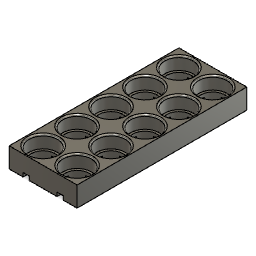
Battery-holder-103.6v-18650 (Autodesk Fusion 360 design; units mm, degrees)
Autodesk Fusion 360 part; units mm, degrees
note: some values were not read from the file. Set by a fixed rule: which sketch regions a step uses.
sketch "Sketch1" plane through (0, 0, 0) normal (0, 1, 0) x (1, 0, 0)
  line L0 (0, 0) -> (-55, 0)
  line L1 (-55, 0) -> (-55, -100.2)
  line L2 (-55, -100.2) -> (0, -100.2)
  line L3 (0, -100.2) -> (0, 0)
  dimension "d1" = 55
  dimension "d2" = 100.2
  constraint horizontal L0
  constraint vertical L1
  constraint horizontal L2
  constraint vertical L3
  constraint coincident L0.start L3.end
  measures "d1" distance of L0.start L0.end
  measures "d2" distance of L0.start L2.end
extrude "Extrude1" add sketch "Sketch1" along normal blind 6
sketch "Sketch2" plane through (0, 6, 0) normal (0, 1, 0) x (-1, 0, 0)
  line L0 (0, 100.2) -> (0, 0)
  line L1 (0, 0) -> (55, 0)
  line L2 (55, 0) -> (55, 100.2)
  line L3 (55, 100.2) -> (0, 100.2)
  circle A0 centre (4, 5) radius 1.5
  circle A1 centre (4, 95.2) radius 1.5
  circle A2 centre (51, 95.2) radius 1.5
  circle A3 centre (51, 5) radius 1.5
  dimension "d13" = 3
  dimension "d14" = 3
  dimension "d15" = 3
  dimension "d16" = 3
  measures "d13" diameter of A0
  measures "d14" diameter of A1
  measures "d15" diameter of A2
  measures "d16" diameter of A3
extrude "Extrude2" cut sketch "Sketch2" against normal blind 6 contours A0 | A1 | A2 | A3
sketch "Sketch3" plane through (0, 6, 0) normal (0, 1, 0) x (-1, 0, 0)
  circle A0 centre (4, 95.2) radius 1.5
  circle A1 centre (51, 5) radius 1.5
  circle A2 centre (51, 95.2) radius 1.5
  circle A3 centre (4, 5) radius 1.5
  line L0 (0, 100.2) -> (0, 0)
  line L1 (0, 0) -> (55, 0)
  line L2 (55, 0) -> (55, 100.2)
  line L3 (55, 100.2) -> (0, 100.2)
  circle A4 centre (4, 95.2) radius 3
  circle A5 centre (51, 95.2) radius 3
  circle A6 centre (4, 5) radius 3
  circle A7 centre (51, 5) radius 3
  dimension "d19" = 1.5
  dimension "d20" = 1.5
  dimension "d21" = 1.5
  dimension "d22" = 1.5
  measures "d19" distance of A0
  measures "d20" distance of A2
  measures "d21" distance of A3
  measures "d22" distance of A1
extrude "Extrude3" add sketch "Sketch3" along normal blind 3 contours A4 | A5 | A6 | A7
extrude "Extrude4" cut 4 faces at (-53.1403, 9, 93.9211) (-6.4832, 9, 4.7764) (-6.1777, 9, 96.4141) (-53.4832, 9, 4.7764) along direction (0, -1, 0) blind 3
sketch "Sketch4" plane through (0, 6, 0) normal (0, 1, 0) x (-1, 0, 0)
  circle A0 centre (4, 95.2) radius 1.5
  circle A1 centre (51, 95.2) radius 1.5
  circle A2 centre (4, 5) radius 1.5
  circle A3 centre (51, 5) radius 1.5
  line L0 (0, 100.2) -> (0, 0)
  line L1 (0, 0) -> (55, 0)
  line L2 (55, 0) -> (55, 100.2)
  line L3 (55, 100.2) -> (0, 100.2)
  circle A4 centre (4, 95.2) radius 1.5
  circle A5 centre (51, 95.2) radius 1.5
  circle A6 centre (51, 5) radius 1.5
  circle A7 centre (4, 5) radius 1.5
  point P0 (2.5, 5)
  constraint concentric A0 A4
  constraint concentric A1 A5
  constraint concentric A3 A6
  constraint concentric A2 A7
  constraint coincident A7 P0
extrude "Extrude5" add sketch "Sketch4" against normal blind 6 contours A0 A4 | A1 A5 | A2 A7 | A3 A6
extrude "Extrude6" cut 1 faces at (0, 2, 66.8) along direction (-1, 0, 0) blind 11
extrude "Extrude7" add 1 faces at (-25.6667, 2, 0) along direction (0, 0, -1) blind 9.8
extrude "Extrude8" add 1 faces at (-25.6667, 6, 63.5333) along direction (0, 1, 0) blind 4.5
sketch "Sketch5" plane through (0, 10.5, 0) normal (0, 1, 0) x (-1, 0, 0)
  line L0 (11, 100.2) -> (11, -9.8)
  line L1 (11, -9.8) -> (55, -9.8)
  line L2 (55, -9.8) -> (55, 100.2)
  line L3 (55, 100.2) -> (11, 100.2)
  line L4 (55, 100.2) -> (33, 100.2)
  line L5 (33, 100.2) -> (33, -9.8)
  line L6 (33, -9.8) -> (55, -9.8)
  line L7 (55, -9.8) -> (55, 100.2)
  line L8 (33, 100.2) -> (11, 100.2)
  line L9 (11, 100.2) -> (11, 78.2)
  line L10 (11, 78.2) -> (33, 78.2)
  line L11 (33, 78.2) -> (33, 100.2)
  line L12 (33, 78.2) -> (55, 78.2)
  line L13 (55, 78.2) -> (55, 56.2)
  line L14 (55, 56.2) -> (33, 56.2)
  line L15 (33, 56.2) -> (33, 78.2)
  line L16 (33, 56.2) -> (11, 56.2)
  line L17 (11, 56.2) -> (11, 34.2)
  line L18 (11, 34.2) -> (33, 34.2)
  line L19 (33, 34.2) -> (33, 56.2)
  line L20 (33, 34.2) -> (55, 34.2)
  line L21 (55, 34.2) -> (55, 12.2)
  line L22 (55, 12.2) -> (33, 12.2)
  line L23 (33, 12.2) -> (33, 34.2)
  line L24 (33, 12.2) -> (11, 12.2)
  line L25 (11, 12.2) -> (11, -9.8)
  line L26 (11, -9.8) -> (33, -9.8)
  line L27 (33, -9.8) -> (33, 12.2)
  circle A0 centre (22, 89.2) radius 9.25
  circle A1 centre (44, 89.2) radius 9.25
  circle A2 centre (44, 67.2) radius 9.25
  circle A3 centre (22, 67.2) radius 9.25
  circle A4 centre (44, 45.2) radius 9.25
  circle A5 centre (22, 45.2) radius 9.25
  circle A6 centre (44, 23.2) radius 9.25
  circle A7 centre (22, 23.2) radius 9.25
  line L28 (33, 12.2) -> (44, 12.2)
  line L29 (44, 12.2) -> (44, 1.2)
  line L30 (44, 1.2) -> (33, 1.2)
  line L31 (33, 1.2) -> (33, 12.2)
  circle A8 centre (44, 1.2) radius 9.25
  line L32 (11, 12.2) -> (22, 12.2)
  line L33 (22, 12.2) -> (22, 1.2)
  line L34 (22, 1.2) -> (11, 1.2)
  line L35 (11, 1.2) -> (11, 12.2)
  circle A9 centre (22, 1.2) radius 9.25
  circle A10 centre (44, 89.2) radius 7.75
  circle A11 centre (44, 67.2) radius 7.75
  circle A12 centre (22, 67.2) radius 7.75
  circle A13 centre (22, 89.2) radius 7.75
  circle A14 centre (44, 45.2) radius 7.75
  circle A15 centre (22, 45.2) radius 7.75
  circle A16 centre (44, 23.2) radius 7.75
  circle A17 centre (22, 23.2) radius 7.75
  circle A18 centre (44, 1.2) radius 7.75
  circle A19 centre (22, 1.2) radius 7.75
  dimension "d35" = 22
  dimension "d36" = 22
  dimension "d37" = 22
  dimension "d38" = 22
  dimension "d39" = 18.5
  dimension "d40" = 18.5
  dimension "d41" = 18.5
  dimension "d42" = 18.5
  dimension "d43" = 18.5
  dimension "d44" = 18.5
  dimension "d45" = 18.5
  dimension "d46" = 18.5
  dimension "d47" = 11
  dimension "d48" = 11
  dimension "d49" = 18.5
  dimension "d50" = 11
  dimension "d51" = 11
  dimension "d52" = 18.5
  dimension "d53" = -1.5
  dimension "d54" = -1.5
  dimension "d55" = -1.5
  dimension "d56" = -1.5
  dimension "d57" = -1.5
  dimension "d58" = -1.5
  dimension "d59" = -1.5
  dimension "d60" = -1.5
  dimension "d61" = -1.5
  dimension "d62" = -1.5
  constraint horizontal L4
  constraint vertical L5
  constraint horizontal L6
  constraint vertical L7
  constraint midpoint L1 L5.end
  constraint coincident L2.end L3.start
  constraint horizontal L8
  constraint vertical L9
  constraint horizontal L10
  constraint vertical L11
  constraint horizontal L12
  constraint vertical L13
  constraint horizontal L14
  constraint vertical L15
  constraint horizontal L16
  constraint vertical L17
  constraint horizontal L18
  constraint vertical L19
  constraint horizontal L20
  constraint vertical L21
  constraint horizontal L22
  constraint vertical L23
  constraint horizontal L24
  constraint vertical L25
  constraint horizontal L26
  constraint vertical L27
  constraint coincident L0.end L1.start
  constraint horizontal L28
  constraint vertical L29
  constraint horizontal L30
  constraint vertical L31
  constraint coincident L29.end L30.start
  constraint horizontal L32
  constraint vertical L33
  constraint horizontal L34
  constraint vertical L35
  constraint coincident L33.end L34.start
  measures "d35" distance of L4.end L10.end
  measures "d36" distance of L10.end L14.end
  measures "d37" distance of L14.end L18.end
  measures "d38" distance of L18.end L22.end
  measures "d39" diameter of A0
  measures "d40" diameter of A1
  measures "d41" diameter of A2
  measures "d42" diameter of A3
  measures "d43" diameter of A4
  measures "d44" diameter of A5
  measures "d45" diameter of A6
  measures "d46" diameter of A7
  measures "d47" distance of L22.end L28.end
  measures "d48" distance of L22.end L30.end
  measures "d49" diameter of A8
  measures "d50" distance of L24.end L32.end
  measures "d51" distance of L24.end L34.end
  measures "d52" diameter of A9
extrude "Extrude9" cut sketch "Sketch5" against normal blind 8.25 contours L33 L34 A9 A19 | L33 L34 A9 A19 | L29 L30 A8 A18 | L29 L30 A8 A18 | A0 | A1 | A2 | A3 | A4 | A5 | A6 | A7
extrude "Extrude10" cut 10 faces at (-41.4455, 10.5, 5.0993) (-20.1623, 10.5, 0.6862) (-23.8937, 10.5, 25.7272) (-41.7934, 10.5, 28.227) (-43.3752, 10.5, 47.3873) (-19.9576, 10.5, 42.7914) (-22.1931, 10.5, 69.4334) (-39.999, 10.5, 68.9366) (-47.0434, 10.5, 90.9571) (-18.5228, 10.5, 88.0791) along direction (0, -1, 0) blind 55
fillet "Fillet1" radius 1 1 edges at (-35.376, 10.5, 4.5449)
fillet "Fillet2" radius 1 1 edges at (-13.376, 10.5, 4.5449)
fillet "Fillet3" radius 1 1 edges at (-35.376, 10.5, 26.5449)
fillet "Fillet4" radius 1 1 edges at (-13.376, 10.5, 26.5449)
fillet "Fillet5" radius 1 1 edges at (-35.376, 10.5, 48.5449)
fillet "Fillet6" radius 1 1 edges at (-13.376, 10.5, 48.5449)
fillet "Fillet7" radius 1 1 edges at (-35.376, 10.5, 70.5449)
fillet "Fillet8" radius 1 1 edges at (-13.376, 10.5, 70.5449)
fillet "Fillet9" radius 1 1 edges at (-35.376, 10.5, 92.5449)
fillet "Fillet10" radius 1 1 edges at (-13.376, 10.5, 92.5449)
extrude "Extrude11" add 1 faces at (-31.2271, 0, 36.1096) along direction (0, -1, 0) blind 1
sketch "Sketch6" plane through (0, -1, 0) normal (0, -1, 0) x (1, 0, 0)
  circle A0 centre (-44, 89.2) radius 7.75
  circle A1 centre (-22, 67.2) radius 7.75
  circle A2 centre (-44, 45.2) radius 7.75
  circle A3 centre (-22, 23.2) radius 7.75
  circle A4 centre (-44, 1.2) radius 7.75
  circle A5 centre (-22, 1.2) radius 7.75
  circle A6 centre (-44, 23.2) radius 7.75
  circle A7 centre (-22, 45.2) radius 7.75
  circle A8 centre (-44, 67.2) radius 7.75
  circle A9 centre (-22, 89.2) radius 7.75
  line L0 (-11, -9.8) -> (-11, 100.2)
  line L1 (-11, 100.2) -> (-55, 100.2)
  line L2 (-55, 100.2) -> (-55, -9.8)
  line L3 (-55, -9.8) -> (-11, -9.8)
  line L4 (-11, 100.2) -> (-33, 100.2)
  line L5 (-33, 100.2) -> (-33, -9.8)
  line L6 (-33, -9.8) -> (-11, -9.8)
  line L7 (-11, -9.8) -> (-11, 100.2)
  line L8 (-33, 100.2) -> (-44, 100.2)
  line L9 (-44, 100.2) -> (-44, -9.8)
  line L10 (-44, -9.8) -> (-33, -9.8)
  line L11 (-33, -9.8) -> (-33, 100.2)
  line L12 (-44, 100.2) -> (-42, 100.2)
  line L13 (-42, 100.2) -> (-42, -9.8)
  line L14 (-42, -9.8) -> (-44, -9.8)
  line L15 (-44, -9.8) -> (-44, 100.2)
  line L16 (-44, 100.2) -> (-46, 100.2)
  line L17 (-46, 100.2) -> (-46, -9.8)
  line L18 (-46, -9.8) -> (-44, -9.8)
  line L19 (-44, -9.8) -> (-44, 100.2)
  line L20 (-11, 100.2) -> (-22, 100.2)
  line L21 (-22, 100.2) -> (-22, -9.8)
  line L22 (-22, -9.8) -> (-11, -9.8)
  line L23 (-11, -9.8) -> (-11, 100.2)
  line L24 (-22, 100.2) -> (-24, 100.2)
  line L25 (-24, 100.2) -> (-24, -9.8)
  line L26 (-24, -9.8) -> (-22, -9.8)
  line L27 (-22, -9.8) -> (-22, 100.2)
  line L28 (-22, -9.8) -> (-20, -9.8)
  line L29 (-20, -9.8) -> (-20, 100.2)
  line L30 (-20, 100.2) -> (-22, 100.2)
  line L31 (-22, 100.2) -> (-22, -9.8)
  line L32 (-11, 100.2) -> (-55, 100.2)
  line L33 (-55, 100.2) -> (-55, 89.2)
  line L34 (-55, 89.2) -> (-11, 89.2)
  line L35 (-11, 89.2) -> (-11, 100.2)
  line L36 (-11, 89.2) -> (-55, 89.2)
  line L37 (-55, 89.2) -> (-55, 87.2)
  line L38 (-55, 87.2) -> (-11, 87.2)
  line L39 (-11, 87.2) -> (-11, 89.2)
  line L40 (-11, 89.2) -> (-55, 89.2)
  line L41 (-55, 89.2) -> (-55, 91.2)
  line L42 (-55, 91.2) -> (-11, 91.2)
  line L43 (-11, 91.2) -> (-11, 89.2)
  line L44 (-55, 67.2) -> (-11, 67.2)
  line L45 (-11, 67.2) -> (-11, 65.2)
  line L46 (-11, 65.2) -> (-55, 65.2)
  line L47 (-55, 65.2) -> (-55, 67.2)
  line L48 (-11, 67.2) -> (-55, 67.2)
  line L49 (-55, 67.2) -> (-55, 69.2)
  line L50 (-55, 69.2) -> (-11, 69.2)
  line L51 (-11, 69.2) -> (-11, 67.2)
  line L52 (-11, 45.2) -> (-55, 45.2)
  line L53 (-55, 45.2) -> (-55, 43.2)
  line L54 (-55, 43.2) -> (-11, 43.2)
  line L55 (-11, 43.2) -> (-11, 45.2)
  line L56 (-11, 45.2) -> (-55, 45.2)
  line L57 (-55, 45.2) -> (-55, 47.2)
  line L58 (-55, 47.2) -> (-11, 47.2)
  line L59 (-11, 47.2) -> (-11, 45.2)
  line L60 (-55, 23.2) -> (-11, 23.2)
  line L61 (-11, 23.2) -> (-11, 21.2)
  line L62 (-11, 21.2) -> (-55, 21.2)
  line L63 (-55, 21.2) -> (-55, 23.2)
  line L64 (-11, 23.2) -> (-55, 23.2)
  line L65 (-55, 23.2) -> (-55, 25.2)
  line L66 (-55, 25.2) -> (-11, 25.2)
  line L67 (-11, 25.2) -> (-11, 23.2)
  line L68 (-55, 1.2) -> (-11, 1.2)
  line L69 (-11, 1.2) -> (-11, -0.8)
  line L70 (-11, -0.8) -> (-55, -0.8)
  line L71 (-55, -0.8) -> (-55, 1.2)
  line L72 (-11, 1.2) -> (-55, 1.2)
  line L73 (-55, 1.2) -> (-55, 3.2)
  line L74 (-55, 3.2) -> (-11, 3.2)
  line L75 (-11, 3.2) -> (-11, 1.2)
  dimension "d89" = 2
  dimension "d90" = 2
  dimension "d91" = 2
  dimension "d92" = 2
  dimension "d93" = 2
  dimension "d94" = 2
  dimension "d95" = 2
  dimension "d96" = 2
  dimension "d97" = 2
  dimension "d98" = 2
  dimension "d99" = 2
  dimension "d100" = 2
  dimension "d101" = 2
  dimension "d102" = 2
  constraint horizontal L4
  constraint vertical L5
  constraint horizontal L6
  constraint vertical L7
  constraint midpoint L3 L5.end
  constraint coincident L0.end L1.start
  constraint horizontal L8
  constraint vertical L9
  constraint horizontal L10
  constraint vertical L11
  constraint coincident L3 L9.end
  constraint horizontal L12
  constraint vertical L13
  constraint horizontal L14
  constraint vertical L15
  constraint horizontal L16
  constraint vertical L17
  constraint horizontal L18
  constraint vertical L19
  constraint horizontal L20
  constraint vertical L21
  constraint horizontal L22
  constraint vertical L23
  constraint midpoint L6 L21.end
  constraint horizontal L24
  constraint vertical L25
  constraint horizontal L26
  constraint vertical L27
  constraint horizontal L28
  constraint vertical L29
  constraint horizontal L30
  constraint vertical L31
  constraint horizontal L32
  constraint vertical L33
  constraint horizontal L34
  constraint vertical L35
  constraint coincident L2 L33.end
  constraint horizontal L36
  constraint vertical L37
  constraint horizontal L38
  constraint vertical L39
  constraint horizontal L40
  constraint vertical L41
  constraint horizontal L42
  constraint vertical L43
  constraint horizontal L44
  constraint vertical L45
  constraint horizontal L46
  constraint vertical L47
  constraint coincident L2 L44.start
  constraint horizontal L48
  constraint vertical L49
  constraint horizontal L50
  constraint vertical L51
  constraint horizontal L52
  constraint vertical L53
  constraint horizontal L54
  constraint vertical L55
  constraint midpoint L23 L52.start
  constraint horizontal L56
  constraint vertical L57
  constraint horizontal L58
  constraint vertical L59
  constraint horizontal L60
  constraint vertical L61
  constraint horizontal L62
  constraint vertical L63
  constraint coincident L2 L60.start
  constraint horizontal L64
  constraint vertical L65
  constraint horizontal L66
  constraint vertical L67
  constraint horizontal L68
  constraint vertical L69
  constraint horizontal L70
  constraint vertical L71
  constraint coincident L2 L68.start
  constraint horizontal L72
  constraint vertical L73
  constraint horizontal L74
  constraint vertical L75
  measures "d89" distance of L8.end L12.end
  measures "d90" distance of L8.end L16.end
  measures "d91" distance of L20.end L24.end
  measures "d92" distance of L21.end L28.end
  measures "d93" distance of L34.end L38.end
  measures "d94" distance of L34.end L42.end
  measures "d95" distance of L44.start L46.end
  measures "d96" distance of L44.end L50.end
  measures "d97" distance of L52.start L54.end
  measures "d98" distance of L52.start L58.end
  measures "d99" distance of L60.start L62.end
  measures "d100" distance of L60.end L66.end
  measures "d101" distance of L68.start L70.end
  measures "d102" distance of L68.end L74.end
extrude "Extrude12" cut sketch "Sketch6" against normal blind 1 contours A0 L5 L11 L34 L36 L38 L40 | A0 L5 L11 L34 L36 L40 L42 | A9 L5 L11 L34 L36 L38 L40 | A9 L5 L11 L34 L36 L40 L42 | A0 A8 L9 L13 L15 L19 | A0 A8 L9 L15 L17 L19 | A1 L5 L11 L44 L48 L50 | A8 L5 L11 L44 L48 L50 | A1 L5 L11 L44 L46 L48 | A8 L5 L11 L44 L46 L48 | A1 A9 L21 L25 L27 L31 | A1 A9 L21 L27 L29 L31 | A7 L5 L11 L52 L56 L58 | A2 L5 L11 L52 L56 L58 | A2 A8 L9 L13 L15 L19 | A7 L5 L11 L52 L54 L56 | A2 L5 L11 L52 L54 L56 | A1 A7 L21 L25 L27 L31 | A2 A8 L9 L15 L17 L19 | A1 A7 L21 L27 L29 L31 | A3 L5 L11 L60 L64 L66 | A6 L5 L11 L60 L64 L66 | A3 L5 L11 L60 L62 L64 | A6 L5 L11 L60 L62 L64 | A2 A6 L9 L13 L15 L19 | A3 A7 L21 L25 L27 L31 | A2 A6 L9 L15 L17 L19 | A3 A7 L21 L27 L29 L31 | A5 L5 L11 L68 L72 L74 | A4 L5 L11 L68 L72 L74 | A5 L5 L11 L68 L70 L72 | A4 L5 L11 L68 L70 L72 | A3 A5 L21 L25 L27 L31 | A4 A6 L9 L13 L15 L19 | A3 A5 L21 L27 L29 L31 | A4 A6 L9 L15 L17 L19
extrude "Extrude13" add 5 faces at (-36.2613, -1, -8.6847) (-31.2916, -1, 80.1818) (-31.2916, -1, 58.1818) (-34.435, -1, 35.9084) (-31.2916, -1, 14.1818) along direction (0, -1, 0) blind 1.5
sketch "Sketch7" plane through (0, -2.5, 0) normal (0, -1, 0) x (1, 0, 0)
  line L0 (-46, 8.6875) -> (-46, 15.7125)
  arc A0 (-46, 30.6875) -> (-46, 15.7125) centre (-44, 23.2) ccw
  line L1 (-46, 30.6875) -> (-46, 37.7125)
  arc A1 (-46, 52.6875) -> (-46, 37.7125) centre (-44, 45.2) ccw
  line L2 (-46, 52.6875) -> (-46, 59.7125)
  arc A2 (-46, 74.6875) -> (-46, 59.7125) centre (-44, 67.2) ccw
  line L3 (-46, 74.6875) -> (-46, 81.7125)
  arc A3 (-36.5125, 91.2) -> (-46, 81.7125) centre (-44, 89.2) ccw
  line L4 (-36.5125, 91.2) -> (-29.4875, 91.2)
  arc A4 (-20, 81.7125) -> (-29.4875, 91.2) centre (-22, 89.2) ccw
  line L5 (-20, 81.7125) -> (-20, 74.6875)
  arc A5 (-20, 59.7125) -> (-20, 74.6875) centre (-22, 67.2) ccw
  line L6 (-20, 59.7125) -> (-20, 52.6875)
  arc A6 (-20, 37.7125) -> (-20, 52.6875) centre (-22, 45.2) ccw
  line L7 (-20, 37.7125) -> (-20, 30.6875)
  arc A7 (-20, 15.7125) -> (-20, 30.6875) centre (-22, 23.2) ccw
  line L8 (-20, 15.7125) -> (-20, 8.6875)
  arc A8 (-29.4875, -0.8) -> (-20, 8.6875) centre (-22, 1.2) ccw
  line L9 (-29.4875, -0.8) -> (-36.5125, -0.8)
  arc A9 (-46, 8.6875) -> (-36.5125, -0.8) centre (-44, 1.2) ccw
  line L10 (-11, -9.8) -> (-11, 100.2)
  line L11 (-11, 100.2) -> (-55, 100.2)
  line L12 (-55, 100.2) -> (-55, -9.8)
  line L13 (-55, -9.8) -> (-11, -9.8)
  line L14 (-22, 100.2) -> (-24, 100.2)
  line L15 (-24, 100.2) -> (-24, -9.8)
  line L16 (-24, -9.8) -> (-22, -9.8)
  line L17 (-22, -9.8) -> (-22, 100.2)
  line L18 (-22, -9.8) -> (-20, -9.8)
  line L19 (-20, -9.8) -> (-20, 100.2)
  line L20 (-20, 100.2) -> (-22, 100.2)
  line L21 (-22, 100.2) -> (-22, -9.8)
  line L22 (-44, 100.2) -> (-46, 100.2)
  line L23 (-46, 100.2) -> (-46, -9.8)
  line L24 (-46, -9.8) -> (-44, -9.8)
  line L25 (-44, -9.8) -> (-44, 100.2)
  line L26 (-44, 100.2) -> (-42, 100.2)
  line L27 (-42, 100.2) -> (-42, -9.8)
  line L28 (-42, -9.8) -> (-44, -9.8)
  line L29 (-44, -9.8) -> (-44, 100.2)
  dimension "d107" = 2
  dimension "d108" = 2
  dimension "d109" = 2
  dimension "d110" = 2
  constraint horizontal L14
  constraint vertical L15
  constraint horizontal L16
  constraint vertical L17
  constraint coincident L11 L14.start
  constraint horizontal L18
  constraint vertical L19
  constraint horizontal L20
  constraint vertical L21
  constraint horizontal L22
  constraint vertical L23
  constraint horizontal L24
  constraint vertical L25
  constraint coincident L11 L22.start
  constraint horizontal L26
  constraint vertical L27
  constraint horizontal L28
  constraint vertical L29
  measures "d107" distance of L14.start L14.end
  measures "d108" distance of L16.end L18.end
  measures "d109" distance of L22.start L22.end
  measures "d110" distance of L22.start L26.end
extrude "Extrude14" cut sketch "Sketch7" against normal blind 2.5 contours A9 L13 L23 L24 L25 L29 | A9 L13 L25 L27 L28 L29 | A3 L11 L25 L26 L27 L29 | A3 L11 L22 L23 L25 L29 | A8 L13 L15 L16 L17 L21 | A4 L11 L14 L15 L17 L21 | A8 L13 L17 L18 L19 L21 | A4 L11 L17 L19 L20 L21
